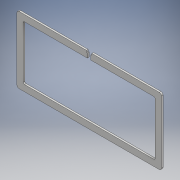
# Autodesk Inventor part: layer4
Saved by Autodesk Inventor 2017 (Build 210142000, 142)
## iProperties
Created: 2021-06-16
Part Number: layer4
Material: Generic
Document SubType Name: Modeling
Designer: Jack
Density: 1 g/cm^3
Appearance: Default
Author: Jack
Autodesk Inventor part; units mm, degrees
ref_plane "YZ Plane" through (0, 0, 0) normal (1, 0, 0) x (0, 1, 0)
ref_plane "XZ Plane" through (0, 0, 0) normal (0, 1, 0) x (-1, 0, 0)
ref_plane "XY Plane" through (0, 0, 0) normal (0, 0, 1) x (1, 0, 0)
sketch "Sketch1" plane through (0, 0, 0) normal (0, 1, 0) x (-1, 0, 0)
  line L0 (-167.3432, 71.9578) -> (-167.3432, -77.8672)
  line L1 (-162.3432, 76.9578) -> (-0.8632, 76.9578)
  line L2 (11.7368, 76.9578) -> (173.2198, 76.9578)
  arc A0 (-162.3432, 76.9578) -> (-167.3432, 71.9578) centre (-162.3432, 71.9578) ccw
  arc A1 (-167.3432, -77.8672) -> (-162.3432, -82.8672) centre (-162.3432, -77.8672) ccw
  line L3 (178.2198, -77.8672) -> (178.2198, 71.9578)
  line L4 (173.2198, -82.8672) -> (-162.3432, -82.8672)
  arc A2 (173.2198, -82.8672) -> (178.2198, -77.8672) centre (173.2198, -77.8672) ccw
  arc A3 (178.2198, 71.9578) -> (173.2198, 76.9578) centre (173.2198, 71.9578) ccw
  line L5 (-149.3552, 61.9583) -> (1.1368, 61.9583)
  line L6 (9.7368, 61.9583) -> (160.2077, 61.9583)
  line L7 (-152.3432, 58.9581) -> (-152.3432, -64.8672)
  line L8 (163.2197, 58.9581) -> (163.2197, -64.8672)
  line L9 (-149.3432, -67.8672) -> (160.2197, -67.8672)
  arc A4 (-149.3432, 61.9583) -> (-152.3432, 58.9289) centre (-149.3432, 58.9581) ccw
  arc A5 (163.2197, 58.9581) -> (160.2077, 61.9583) centre (160.3139, 59.0529) ccw
  arc A6 (160.2197, -67.8672) -> (163.2197, -64.8672) centre (160.2197, -64.8672) ccw
  arc A7 (-152.3432, -64.8672) -> (-149.3432, -67.8672) centre (-149.3432, -64.8672) ccw
  line L10 (1.1368, 72.9578) -> (1.1368, 61.9583)
  line L11 (9.7368, 72.9578) -> (9.7368, 61.9583)
  line L12 (1.1368, 72.9578) -> (-0.8632, 72.9578)
  line L13 (9.7368, 72.9578) -> (11.7368, 72.9578)
  line L14 (11.7368, 72.9578) -> (11.7368, 76.9578)
  line L15 (-0.8632, 72.9578) -> (-0.8632, 76.9578)
  point P0 (0, 0)
  constraints: 32 end point, 16 point on circle, 8 centre point, 2 point on line
extrude "Extrusion1" add sketch "Sketch1" along normal blind 4
body "Solid1"
